Spielzeugzug_verbinder_v2 (Autodesk Fusion 360 design; units mm, degrees)
Autodesk Fusion 360 part; units mm, degrees
sketch "Sketch1" plane through (0, 0, 0) normal (0, 1, 0) x (1, 0, 0)
  circle A0 centre (0, 0) radius 5.65
  circle A1 centre (23.5, 0) radius 5.65
  line L0 (19.8818, 3.05) -> (4.1182, 3.05)
  line L1 (4.1182, 3.05) -> (4.1182, -3.05)
  line L2 (4.1182, -3.05) -> (19.8818, -3.05)
  line L3 (19.8818, -3.05) -> (19.8818, 3.05)
  line L4 (19.8818, 3.05) -> (4.1182, -3.05) construction
  line L5 (4.1182, 3.05) -> (19.8818, -3.05) construction
  point P0 (12, 0)
  dimension "d1" = 11.3
  dimension "d2" = 11.3
  dimension "d3" = 6.1
  constraint coincident A0.centre origin
  constraint horizontal L0
  constraint perpendicular L0 L1
  constraint parallel L0 L2
  constraint parallel L1 L3
  constraint coincident L4 P0
  constraint coincident L5 P0
  measures "d1" diameter of A0
  measures "d2" diameter of A1
  measures "d3" distance of L0.end L1.end
extrude "Extrude1" add sketch "Sketch1" along normal blind 12.1
fillet "Fillet1" radius 1.5 4 edges at (-5.65, 12.1, 0) (11.75, 12.1, 3.05) (11.75, 12.1, -3.05) (29.15, 12.1, 0)
fillet "Fillet2" radius 1 4 edges at (11.75, 0, 3.05) (-5.65, 0, 0) (29.15, 0, 0) (11.75, 0, -3.05)
fillet "Fillet3" radius 2 12 edges at (4.5782, 0.2675, 2.7307) (4.756, 5.8, 3.05) (4.4839, 11.7032, 2.5664) (18.9218, 0.2675, 2.7307) (18.744, 5.8, 3.05) (19.0161, 11.7032, 2.5664) (18.9218, 0.2675, -2.7307) (18.744, 5.8, -3.05) (19.0161, 11.7032, -2.5664) (4.5782, 0.2675, -2.7307) (4.756, 5.8, -3.05) (4.4839, 11.7032, -2.5664)
